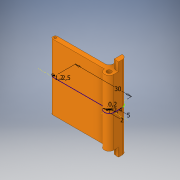
# Autodesk Inventor part: Bottom-Lip
Saved by Autodesk Inventor 2018.3 (Build 223284000, 284)
## iProperties
Created: 2018-05-20
Part Number: Bottom-Lip
Material: Generisch
Document SubType Name: Modeling
Designer: JochenAlt
Density: 1 g/cm^3
Appearance: Orange
Author: JochenAlt
Autodesk Inventor part; units mm, degrees
ref_plane "YZ Plane" through (0, 0, 0) normal (1, 0, 0) x (0, 1, 0)
ref_plane "XZ Plane" through (0, 0, 0) normal (0, 1, 0) x (-1, 0, 0)
ref_plane "XY Plane" through (0, 0, 0) normal (0, 0, 1) x (1, 0, 0)
sketch "Skizze1" plane through (0, 0, 0) normal (0, 0, 1) x (1, 0, 0)
  line L0 (0, 9.4989) -> (0, -4.4998) construction
  line L1 (-38.1036, 0) -> (9.8713, 0) construction
  circle A0 centre (0, 0) radius 2.5
  arc A1 (-30, 2.5) -> (-30, 0) centre (-30, 1.25) ccw
  line L2 (-30, 2.5) -> (-4.5, 2.5)
  line L3 (-30, 0) -> (-2.5, 0)
  circle A2 centre (0, 0) radius 1.2
  circle A3 centre (-30, 1.25) radius 0.6
  circle A4 centre (-30, 1.25) radius 1.25
  line L4 (0, 2.5) -> (0, 6.9813)
  arc A5 (2.5, 4.4813) -> (0, 6.9813) centre (0, 4.4813) ccw
  line L5 (2.5, 2.5) -> (2.5, 0)
  line L6 (1.0198, 2.5) -> (2.5, 2.5)
  line L7 (2.5, 2.5) -> (2.5, 4.4813)
  arc A6 (0, 6.9813) -> (-2.5, 4.4813) centre (0, 4.4813) ccw
  line L8 (-2.5, 4.4813) -> (-2.5, 4.5)
  arc A7 (-4.5, 2.5) -> (-2.5, 4.5) centre (-4.5, 4.5) ccw
  arc A8 (1.0198, 2.5) -> (0, 2.7) centre (0, 0) ccw
  point P0 (-2.5, 0)
  dimension "d0" = 5
  dimension "d1" = 2.5
  dimension "d3" = 2.4
  dimension "d6" = 30
  dimension "d12" = 1.2
  dimension "d21" = 2
  dimension "d22" = 0.2
  constraints: 14 end point, 14 point on circle, 9 tangent, 8 centre point, 5 coincident, 4 point on line, 3 horizontal, 2 equal radius, 1 concentric, 1 line through centre, 1 parallel, 1 vertical, 1 vertical alignment, 2 other
  measures "d0" diameter of A0
  measures "d1" diameter of A1
  measures "d3" diameter of A2
  measures "d6" distance from line of L0 A1.centre
  measures "d12" diameter of A3
  measures "d21" radius of A7
  measures "d22" radial gap between concentric circles of A8 A0
extrude "Extrusion1" add sketch "Skizze1" along normal mid plane 35 contours A0 | A0 L4 A8 L6 L5 | A0 L3 A4 L2 A7 A6 L4 | A1 A4
extrude "Extrusion6" add sketch "Skizze1" along normal mid plane 44 contours L6 A8 L4 A5 L7
